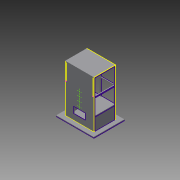
# Autodesk Inventor part: NRCC_Facade
Saved by Autodesk Inventor 2013 SP2 (Build 170200200, 200)
## iProperties
Created: 2010-07-22
Part Number: NRCC_Facade
Document SubType Name: Modeling
Designer: sbareham
Density: 1 g/cm^3
Material: Generic
Author: sbareham
Autodesk Inventor part; units mm, degrees
ref_plane "YZ Plane" through (0, 0, 0) normal (1, 0, 0) x (0, 1, 0)
ref_plane "XZ Plane" through (0, 0, 0) normal (0, 1, 0) x (-1, 0, 0)
ref_plane "XY Plane" through (0, 0, 0) normal (0, 0, 1) x (1, 0, 0)
sketch "Sketch1" plane through (0, 0, 0) normal (0, 0, 1) x (1, 0, 0)
  line L0 (-4178, 3403) -> (4178, 3403)
  line L1 (4178, 3403) -> (4178, -3403)
  line L2 (4178, -3403) -> (-4178, -3403)
  line L3 (-4178, -3403) -> (-4178, 3403)
  line L4 (-3178, 2403) -> (3178, 2403)
  line L5 (3178, 2403) -> (3178, -2403)
  line L6 (3178, -2403) -> (-3178, -2403)
  line L7 (-3178, -2403) -> (-3178, 2403)
  point P0 (0, 0)
  point P1 (4178, 0)
  point P2 (0, 3403)
  dimension "d0" = 8356
  dimension "d1" = 6806
  dimension "d2" = 1000
  dimension "d3" = 1000
  dimension "d4" = 1000
  dimension "d60" = 1000
  constraints: 16 end point, 4 parallel, 2 horizontal, 2 midpoint, 2 perpendicular, 1 horizontal alignment, 1 vertical alignment
  measures "d0" distance between parallel lines of L1 L3
  measures "d1" distance between parallel lines of L0 L2
  measures "d2" distance between parallel lines of L0 L4
  measures "d3" distance between parallel lines of L1 L5
  measures "d4" distance between parallel lines of L3 L7
  measures "d60" distance between parallel lines of L2 L6
extrude "Extrusion7" add sketch "Sketch1" along normal blind 10706 contours L4 L5 L6 L7
shell "Shell1" thickness 203 removed faces 1 at (-1059.3333, 801, 0)
extrude "Extrusion8" add sketch "Sketch1" along normal blind 203 contours L0 L1 L2 L3 | L4 L5 L6 L7
sketch "Sketch5" plane through (3178, -2403, 10706) normal (1, 0, 0) x (0, 0, -1)
  line L0 (10503, 0) -> (10503, 4806) projected
  line L1 (10503, 4806) -> (0, 4806) projected
  line L2 (0, 4806) -> (0, 0) projected
  line L3 (10503, 0) -> (0, 0) projected
  line L4 (203, 203) -> (3876.5, 203)
  line L5 (3876.5, 203) -> (3876.5, 4603)
  line L6 (3876.5, 4603) -> (203, 4603)
  line L7 (203, 4603) -> (203, 203)
  line L8 (4079.5, 203) -> (7753, 203)
  line L9 (7753, 203) -> (7753, 4603)
  line L10 (7753, 4603) -> (4079.5, 4603)
  line L11 (4079.5, 4603) -> (4079.5, 203)
  line L12 (7753, 203) -> (10503, 203)
  line L13 (10503, 203) -> (10503, 4603)
  line L14 (10503, 4603) -> (7753, 4603)
  line L15 (7753, 4603) -> (7753, 203)
  line L16 (203, 4603) -> (203, 203) projected
  point P0 (10706, 2403)
  dimension "d66" = 203
  dimension "d67" = 203
  dimension "d68" = 2750
  dimension "d70" = 10300
  dimension "d71" = 3673.5
  dimension "d72" = 3673.5
  dimension "d73" = 203
  dimension "d115" = 203
  constraints: 24 end point, 6 collinear, 6 parallel, 3 horizontal, 3 perpendicular
  measures "d66" distance between parallel lines of L3 L12
  measures "d67" distance between parallel lines of L1 L14
  measures "d68" distance between parallel lines of L0 L15
  measures "d70" distance between parallel lines of L13 L16
  measures "d71" distance between parallel lines of L11 L9
  measures "d72" distance between parallel lines of L7 L5
  measures "d73" distance between parallel lines of L2 L7
  measures "d115" distance between parallel lines of L5 L11
extrude "Extrusion9" cut sketch "Sketch5" against normal blind 6356 contours L8 L11 L10 L9 | L7 L6 L5 L4
sketch "Sketch6" plane through (-3178, 2403, 10706) normal (0, 1, 0) x (1, 0, 0)
  line L0 (6356, 10503) -> (0, 10503) projected
  line L1 (0, 10503) -> (0, 0) projected
  line L2 (6356, 10503) -> (6356, 0) projected
  line L3 (6153, 203) -> (3279.5, 203)
  line L4 (3279.5, 203) -> (3279.5, 3775)
  line L5 (3279.5, 3775) -> (6153, 3775)
  line L6 (6153, 3775) -> (6153, 203)
  line L7 (3076.5, 203) -> (203, 203)
  line L8 (203, 203) -> (203, 3775)
  line L9 (203, 3775) -> (3076.5, 3775)
  line L10 (3076.5, 3775) -> (3076.5, 203)
  line L11 (6153, 3978) -> (3279.5, 3978)
  line L12 (3279.5, 3978) -> (3279.5, 7550)
  line L13 (3279.5, 7550) -> (6153, 7550)
  line L14 (6153, 7550) -> (6153, 3978)
  line L15 (3076.5, 3978) -> (203, 3978)
  line L16 (203, 3978) -> (203, 7550)
  line L17 (203, 7550) -> (3076.5, 7550)
  line L18 (3076.5, 7550) -> (3076.5, 3978)
  line L19 (6153, 7550) -> (203, 7550)
  line L20 (203, 7550) -> (203, 10503)
  line L21 (203, 10503) -> (6153, 10503)
  line L22 (6153, 10503) -> (6153, 7550)
  line L23 (203, 10503) -> (6153, 10503) projected
  line L24 (6356, 203) -> (0, 203) projected
  line L25 (0, 0) -> (6356, 0) projected
  point P0 (3178, 10706)
  dimension "d77" = 203
  dimension "d78" = 203
  dimension "d79" = 2953
  dimension "d82" = 5950
  dimension "d83" = 2873.5
  dimension "d84" = 2873.5
  dimension "d85" = 203
  dimension "d86" = 7347
  dimension "d87" = 3572
  dimension "d88" = 3572
  dimension "d110" = 10300
  dimension "d111" = 203
  dimension "d112" = 203
  constraints: 40 end point, 13 collinear, 10 parallel, 5 horizontal, 5 perpendicular
  measures "d77" distance between parallel lines of L2 L22
  measures "d78" distance between parallel lines of L1 L20
  measures "d79" distance between parallel lines of L19 L0
  measures "d82" distance between parallel lines of L16 L14
  measures "d83" distance between parallel lines of L12 L14
  measures "d84" distance between parallel lines of L16 L18
  measures "d85" distance between parallel lines of L18 L12
  measures "d86" distance between parallel lines of L24 L13
  measures "d87" distance between parallel lines of L11 L13
  measures "d88" distance between parallel lines of L3 L5
  measures "d110" distance between parallel lines of L23 L7
  measures "d111" distance between parallel lines of L11 L5
  measures "d112" distance between parallel lines of L25 L24
extrude "Extrusion10" cut sketch "Sketch6" against normal blind 203 contours L14 L11 L12 L13 | L3 L4 L5 L6 | L17 L18 L15 L16 | L7 L8 L9 L10
sketch "Sketch7" plane through (-3178, -2403, 10706) normal (0, -1, 0) x (1, 0, 0)
  line L0 (0, -10503) -> (6356, -10503) projected
  line L1 (6356, -10503) -> (6356, 0) projected
  line L2 (0, -10503) -> (0, 0) projected
  line L3 (1878, -7803) -> (4478, -7803)
  line L4 (4478, -7803) -> (4478, -9173)
  line L5 (4478, -9173) -> (1878, -9173)
  line L6 (1878, -9173) -> (1878, -7803)
  line L7 (6153, -203) -> (6153, -3775) projected
  line L8 (203, -3775) -> (203, -203) projected
  point P0 (3178, -10706)
  point P1 (6153, -3775)
  point P2 (3178, -7303)
  point P3 (3178, -6303)
  point P4 (3178, -5303)
  point P5 (3178, -4303)
  dimension "d91" = 1370
  dimension "d92" = 2600
  dimension "d93" = 5950
  dimension "d94" = 1878
  dimension "d95" = 1878
  dimension "d96" = 2700
  dimension "d97" = 500
  dimension "d98" = 1000
  dimension "d99" = 1000
  dimension "d100" = 1000
  constraints: 8 end point, 2 parallel, 1 horizontal, 1 perpendicular
  measures "d91" distance between parallel lines of L3 L5
  measures "d92" distance between parallel lines of L4 L6
  measures "d93" distance between parallel lines of L7 L8
  measures "d94" distance between parallel lines of L2 L6
  measures "d95" distance between parallel lines of L1 L4
  measures "d96" distance between parallel lines of L0 L3
  measures "d97" distance from line of point (3178, -7303) L3
  measures "d98" distance of point (3178, -6303) point (3178, -7303)
  measures "d99" distance of point (3178, -5303) point (3178, -6303)
  measures "d100" distance of point (3178, -5303) point (3178, -4303)
hole "Hole2" at (0, -2403, 3403) at (0, -2403, 4403) at (0, -2403, 5403) at (0, -2403, 6403) direction (0, 1, 0) diameter 125 depth 203 tip angle 118
extrude "Extrusion11" cut sketch "Sketch7" against normal blind 203
extrude "Extrusion14" add sketch "Sketch1" along normal up to surface (203 mm away) from surface at 2953 contours L4 L5 L6 L7
body "Solid2"
